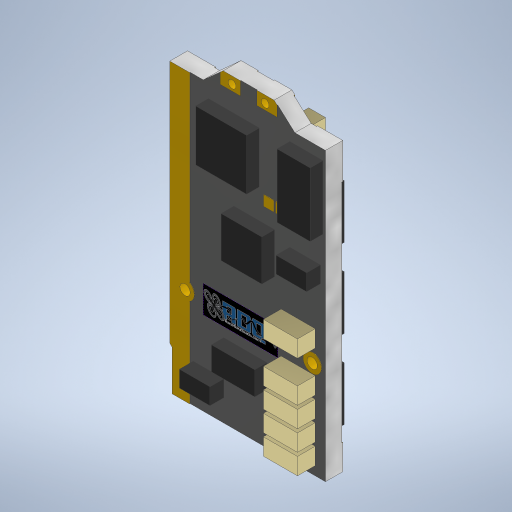
# Autodesk Inventor part: RDQ ESC32
Saved by Autodesk Inventor 2023.1 (Build 271208000, 208)
## iProperties
Created: 2022-10-08
Part Number: RDQ ESC32
Material: GFRC
Document SubType Name: Modeling
Designer: Nathan Cai
Density: 1.7 g/cm^3
Appearance: Flat - Polished Gray
Mass: 3.56 g
Surface Area: 10.1161 cm^2
Volume: 0.696974 cm^3
Author: Nathan Cai
Autodesk Inventor part; units mm, degrees
ref_plane "YZ Plane" through (0, 0, 0) normal (1, 0, 0) x (0, 1, 0)
ref_plane "XZ Plane" through (0, 0, 0) normal (0, 1, 0) x (-1, 0, 0)
ref_plane "XY Plane" through (0, 0, 0) normal (0, 0, 1) x (1, 0, 0)
sketch "Sketch1" plane through (0, 0, 0) normal (0, 0, 1) x (1, 0, 0)
  line L0 (-7.5, 15) -> (7.5, 15)
  line L1 (7.5, 15) -> (7.5, -15)
  line L2 (7.5, -15) -> (-7.5, -15)
  line L3 (-7.5, -15) -> (-7.5, 15)
  line L4 (-7.5, 15) -> (7.5, -15) construction
  line L5 (7.5, 15) -> (-7.5, -15) construction
  line L6 (-7.5, 13.2) -> (7.5, 13.2)
  line L7 (-2.5, 11.4) -> (2.5, 11.4) construction
  line L8 (2.5, 11.4) -> (2.5, 15) construction
  line L9 (2.5, 15) -> (-2.5, 15)
  line L10 (-2.5, 15) -> (-2.5, 11.4) construction
  line L11 (-2.5, 11.4) -> (2.5, 15) construction
  line L12 (2.5, 11.4) -> (-2.5, 15) construction
  line L13 (-4.5, 13.2) -> (-2.5, 15)
  line L14 (2.5, 15) -> (4.5, 13.2)
  line L15 (-4.5, 13.2) -> (4.5, 13.2) construction
  point P0 (0, 0)
  point P1 (0, 13.2)
  dimension "d0" = 15
  dimension "d1" = 30
  dimension "d4" = 28.2
  dimension "d5" = 5
  dimension "d6" = 9
  constraints: 32 end point, 6 midpoint, 5 point on line, 4 parallel, 3 perpendicular, 2 horizontal, 1 collinear
  measures "d0" distance of L1.end L2.end
  measures "d1" distance of L0.end L1.end
  measures "d4" distance between parallel lines of L2 L6
  measures "d5" distance of L9.end L8.end
  measures "d6" distance of L14.end L13.start
extrude "Extrusion1" add sketch "Sketch1" along normal blind 1.6 contours L0 L14 L6 L13 | L6 L1 L2 L3
sketch "Sketch3" plane through (0, 0, 1.6) normal (0, 0, 1) x (1, 0, 0)
  line L0 (2.5, 15) -> (-2.5, 15) projected
  line L1 (-0.8, 15) -> (-2.8, 15)
  line L2 (-2.8, 15) -> (-2.8, 13.7)
  line L3 (-2.8, 13.7) -> (-0.8, 13.7)
  line L4 (-0.8, 13.7) -> (-0.8, 15)
  line L5 (2.5, 15) -> (-2.5, 15) projected
  line L6 (0, 15) -> (0, -15) construction
  line L7 (-7.5, -15) -> (7.5, -15) projected
  line L8 (0.8, 15) -> (2.8, 15)
  line L9 (2.8, 15) -> (2.8, 13.7)
  line L10 (2.8, 13.7) -> (0.8, 13.7)
  line L11 (0.8, 13.7) -> (0.8, 15)
  line L12 (-4.5, 13.2) -> (-7.5, 13.2) projected
  line L13 (-7.5, 13.2) -> (-5.8, 13.2)
  line L14 (-5.8, -15) -> (-7.5, -15)
  line L15 (-7.5, -15) -> (-7.5, 13.2)
  circle A0 centre (-6.25, -5.5) radius 0.5
  circle A1 centre (-6.25, -5.5) radius 0.9
  circle A2 centre (6.25, -5.5) radius 0.5
  circle A3 centre (6.25, -5.5) radius 0.9
  line L16 (-5.8, 13.2) -> (-5.8, -4.7206)
  line L17 (-5.8, -6.2794) -> (-5.8, -15)
  line L18 (1.45, 6.45) -> (2.45, 6.45)
  line L19 (2.45, 6.45) -> (2.45, 5.45)
  line L20 (2.45, 5.45) -> (1.45, 5.45)
  line L21 (1.45, 5.45) -> (1.45, 6.45)
  line L22 (1.45, 6.45) -> (2.45, 5.45) construction
  line L23 (2.45, 6.45) -> (1.45, 5.45) construction
  line L24 (2.65, 5.45) -> (3.65, 5.45)
  line L25 (3.65, 5.45) -> (3.65, 6.45)
  line L26 (3.65, 6.45) -> (2.65, 6.45)
  line L27 (2.65, 6.45) -> (2.65, 5.45)
  line L28 (2.65, 5.45) -> (3.65, 6.45) construction
  line L29 (3.65, 5.45) -> (2.65, 6.45) construction
  line L30 (7.5, 13.2) -> (4.5, 13.2) projected
  line L31 (7.5, -15) -> (7.5, 13.2) projected
  circle A4 centre (-1.625, 14.3) radius 0.375
  circle A5 centre (1.625, 14.3) radius 0.375
  line L32 (-7.5, 13.2) -> (-7.5, -15) projected
  line L33 (-7.5, 13.2) -> (-7.75, 13.2)
  line L34 (-7.75, 13.2) -> (-7.75, -10.8)
  line L35 (-7.75, -10.8) -> (-7.5, -10.8) construction
  line L36 (-7.5, -10.8) -> (-7.5, 13.2)
  line L37 (-7.75, -10.8) -> (-7.4606, -11.0894)
  line L38 (-7.75, -10.8) -> (-7.3407, -10.8) construction
  line L39 (-4.5, 13.2) -> (-2.5, 15)
  line L40 (2.5, 15) -> (4.5, 13.2)
  point P0 (0, 0)
  point P1 (-2.8, 14.35)
  point P2 (1.95, 5.95)
  point P3 (3.15, 5.95)
  point P4 (-7.5, -11.05)
  point P5 (2.8, 14.73)
  point P6 (-2.8, 14.73)
  dimension "d8" = 2
  dimension "d9" = 1.3
  dimension "d10" = 5.6
  dimension "d11" = 1.7
  dimension "d12" = 1
  dimension "d13" = 1.25
  dimension "d14" = 1.8
  dimension "d15" = 9.5
  dimension "d16" = 1
  dimension "d17" = 1
  dimension "d18" = 1
  dimension "d19" = 1
  dimension "d20" = 0.2
  dimension "d21" = 6.75
  dimension "d22" = 3.85
  dimension "d23" = 0.75
  dimension "d24" = 3.25
  dimension "d25" = 0.7
  dimension "d28" = 0.25
  dimension "d29" = 24
  dimension "d30" = 45
  constraints: 68 end point, 11 parallel, 7 midpoint, 7 symmetric about line, 6 centre point, 6 horizontal, 6 perpendicular, 4 point on line, 2 coincident, 2 point on circle, 1 equal length, 3 other
  measures "d8" distance of L3.end L2.end
  measures "d9" distance of L2.end L1.end
  measures "d10" distance from line of point (-2.8, 14.35) L9
  measures "d11" distance of L14.start L14.end
  measures "d12" diameter of A0
  measures "d13" distance from line of L15 A0.centre
  measures "d14" diameter of A1
  measures "d15" distance from line of L7 A1.centre
  measures "d16" distance of L19.end L20.end
  measures "d17" distance of L18.end L19.end
  measures "d18" distance of L26.end L25.end
  measures "d19" distance of L25.end L24.end
  measures "d20" distance between parallel lines of L19 L27
  measures "d21" distance between parallel lines of L30 L26
  measures "d22" distance between parallel lines of L31 L25
  measures "d23" diameter of A4
  measures "d24" distance between centres of A4 A5
  measures "d25" distance from line of L0 A4.centre
  measures "d28" distance of L35.end L34.end
  measures "d29" distance of L34.end L33.end
  measures "d30" angle of L37 L38
extrude "Extrusion2" add sketch "Sketch3" along normal blind 0.05 contours L40 L9 L10 L11 L0 | L4 L3 L2 L39 L0 | L7 L15 L12 L16 A1 L17 | A1 | A3 | L18 L19 L20 L21 | L27 L26 L25 L24
extrude "Extrusion3" add sketch "Sketch3" along normal blind 0.05 and the other way blind 1.6 contours L15 L37 L34 L33
extrude "Extrusion4" cut sketch "Sketch3" against normal through all contours A0 | A2 | A4 | A5
extrude "Extrusion5" add sketch "Sketch3" against normal blind 1.7 contours L40 L9 L10 L11 L0 | L4 L3 L2 L39 L0 | A1 | A3
sketch "Sketch4" plane through (0, 0, 0) normal (0, 0, -1) x (-1, 0, 0)
  line L0 (7.5, -11.05) -> (7.75, -10.8) projected
  line L1 (4.5, 13.2) -> (7.75, 13.2) projected
  line L2 (7.5, -11.05) -> (7.75, -11.05) construction
  line L3 (7.75, -11.05) -> (7.75, 13.2)
  line L4 (7.75, 13.2) -> (7.5, 13.2)
  line L5 (7.5, 13.2) -> (7.5, -11.05)
  line L6 (7.5, -11.05) -> (7.75, -10.8)
  line L7 (-7.5, -15) -> (-7.5, 13.2) projected
  line L8 (-7.5, 13.2) -> (-5, 13.2)
  line L9 (-5, 13.2) -> (-5, 9.7)
  line L10 (-5, 9.7) -> (-7.5, 9.7)
  line L11 (-7.5, 9.7) -> (-7.5, 13.2)
  line L12 (7.5, 13.2) -> (5, 13.2)
  line L13 (5, 13.2) -> (5, 9.7)
  line L14 (5, 9.7) -> (7.5, 9.7)
  line L15 (7.5, 9.7) -> (7.5, 13.2)
  line L16 (-7.5, -15) -> (-4.1, -15)
  line L17 (-4.1, -15) -> (-4.1, -12.5)
  line L18 (-4.1, -12.5) -> (-7.5, -12.5)
  line L19 (-7.5, -12.5) -> (-7.5, -15)
  line L20 (7.5, -15) -> (-7.5, -15) projected
  line L21 (7.5, -15) -> (4, -15)
  line L22 (4, -15) -> (4, -12.5)
  line L23 (4, -12.5) -> (7.5, -12.5)
  line L24 (7.5, -12.5) -> (7.5, -15)
  line L25 (-2.1, -15) -> (1.4, -15)
  line L26 (1.4, -15) -> (1.4, -12.5)
  line L27 (1.4, -12.5) -> (-2.1, -12.5)
  line L28 (-2.1, -12.5) -> (-2.1, -15)
  point P0 (0, 0)
  point P1 (1.4, -15)
  dimension "d39" = 2.5
  dimension "d40" = 3.5
  dimension "d41" = 2.5
  dimension "d42" = 3.5
  dimension "d43" = 3.4
  dimension "d44" = 2.5
  dimension "d45" = 3.5
  dimension "d46" = 2.5
  dimension "d47" = 3.5
  dimension "d48" = 2.5
  dimension "d49" = 2
  constraints: 50 end point, 13 equal length, 6 horizontal, 6 perpendicular, 1 point on line
  measures "d39" distance of L9.end L10.end
  measures "d40" distance of L8.end L9.end
  measures "d41" distance of L14.end L13.end
  measures "d42" distance of L13.end L12.end
  measures "d43" distance of L18.end L17.end
  measures "d44" distance of L17.end L16.end
  measures "d45" distance of L22.end L23.end
  measures "d46" distance of L21.end L22.end
  measures "d47" distance of L27.end L26.end
  measures "d48" distance of L26.end L25.end
  measures "d49" distance between parallel lines of L17 L28
extrude "Extrusion6" add sketch "Sketch4" along normal blind 0.1
sketch "Sketch5" plane through (0, 0, 0) normal (0, 0, -1) x (-1, 0, 0)
  line L0 (-0.75, 8.7) -> (-6.5, 8.7)
  line L1 (-6.5, 8.7) -> (-6.5, 3.45)
  line L2 (-6.5, 3.45) -> (-0.75, 3.45)
  line L3 (-0.75, 3.45) -> (-0.75, 8.7)
  line L4 (-7.5, -12.5) -> (-7.5, 9.7) projected
  line L5 (-7.5, 9.7) -> (-5, 9.7) projected
  line L6 (-0.75, 0.95) -> (-6.5, 0.95)
  line L7 (-6.5, 0.95) -> (-6.5, -4.3)
  line L8 (-6.5, -4.3) -> (-0.75, -4.3)
  line L9 (-0.75, -4.3) -> (-0.75, 0.95)
  line L10 (-0.75, -6.8) -> (-6.5, -6.8)
  line L11 (-6.5, -6.8) -> (-6.5, -12.05)
  line L12 (-6.5, -12.05) -> (-0.75, -12.05)
  line L13 (-0.75, -12.05) -> (-0.75, -6.8)
  line L14 (6, 8.7) -> (0.25, 8.7)
  line L15 (0.25, 8.7) -> (0.25, 3.45)
  line L16 (0.25, 3.45) -> (6, 3.45)
  line L17 (6, 3.45) -> (6, 8.7)
  line L18 (6, 0.95) -> (0.25, 0.95)
  line L19 (0.25, 0.95) -> (0.25, -4.3)
  line L20 (0.25, -4.3) -> (6, -4.3)
  line L21 (6, -4.3) -> (6, 0.95)
  line L22 (6, -6.8) -> (0.25, -6.8)
  line L23 (0.25, -6.8) -> (0.25, -12.05)
  line L24 (0.25, -12.05) -> (6, -12.05)
  line L25 (6, -12.05) -> (6, -6.8)
  line L26 (-1.15, 12.7) -> (2.25, 12.7)
  line L27 (2.25, 12.7) -> (2.25, 9.3)
  line L28 (2.25, 9.3) -> (-1.15, 9.3)
  line L29 (-1.15, 9.3) -> (-1.15, 12.7)
  line L30 (-1.15, 12.7) -> (2.25, 9.3) construction
  line L31 (2.25, 12.7) -> (-1.15, 9.3) construction
  line L32 (7.75, 13.2) -> (5, 13.2) projected
  point P0 (0, 0)
  point P1 (0.55, 11)
  dimension "d52" = 5.25
  dimension "d53" = 5.75
  dimension "d54" = 1
  dimension "d55" = 1
  dimension "d65" = 7.75
  dimension "d68" = 6.75
  dimension "d71" = 3.4
  dimension "d72" = 3.4
  dimension "d73" = 6.35
  dimension "d74" = 0.5
  constraints: 60 end point, 4 parallel, 3 horizontal, 2 collinear, 2 midpoint, 2 perpendicular, 1 vertical, 38 other
  measures "d52" distance between parallel lines of L0 L2
  measures "d53" distance of L1.end L2.end
  measures "d54" distance between parallel lines of L4 L1
  measures "d55" distance between parallel lines of L5 L0
  measures "d65" distance of L0.start L6.start
  measures "d68" distance of L0.start L14.start
  measures "d71" distance of L27.end L28.end
  measures "d72" distance of L26.end L27.end
  measures "d73" distance between parallel lines of L4 L29
  measures "d74" distance between parallel lines of L32 L26
extrude "Extrusion7" add sketch "Sketch5" along normal blind 1.25
sketch "Sketch6" plane through (0, 0, -1.25) normal (0, 0, -1) x (-1, 0, 0)
  line L0 (-1.15, 12.7) -> (2.25, 12.7) projected
  line L1 (0.55, 12.7) -> (0.55, 9.3) construction
  line L2 (-1.15, 9.3) -> (2.25, 9.3) projected
  circle A0 centre (0.55, 11) radius 1.375
  point P0 (0, 0)
  dimension "d77" = 2.75
  constraints: 3 midpoint, 2 end point, 1 centre point
  measures "d77" diameter of A0
extrude "Extrusion8" cut sketch "Sketch6" against normal blind 0.1
chamfer "Chamfer1" distance 0.1 angle 45 1 edges at (0.825, 11, -1.15)
sketch "Sketch7" plane through (0, 0, 0) normal (0, 0, -1) x (-1, 0, 0)
  line L0 (-4.15, 12.65) -> (-2.5, 12.65)
  line L1 (-2.5, 12.65) -> (-2.5, 9.3)
  line L2 (-2.5, 9.3) -> (-4.15, 9.3)
  line L3 (-4.15, 9.3) -> (-4.15, 12.65)
  line L4 (-4.15, 12.65) -> (-2.5, 9.3) construction
  line L5 (-2.5, 12.65) -> (-4.15, 9.3) construction
  line L6 (-7.5, 13.2) -> (-7.5, 9.7) projected
  line L7 (-4.1, 2.95) -> (-0.75, 2.95)
  line L8 (-0.75, 2.95) -> (-0.75, 1.3)
  line L9 (-0.75, 1.3) -> (-4.1, 1.3)
  line L10 (-4.1, 1.3) -> (-4.1, 2.95)
  line L11 (-4.1, 2.95) -> (-0.75, 1.3) construction
  line L12 (-0.75, 2.95) -> (-4.1, 1.3) construction
  line L13 (-7.5, -12.5) -> (-7.5, 9.7) projected
  line L14 (-6.5, 3.45) -> (-0.75, 3.45) projected
  line L15 (-4.1, -4.8) -> (-0.75, -4.8)
  line L16 (-0.75, -4.8) -> (-0.75, -6.45)
  line L17 (-0.75, -6.45) -> (-4.1, -6.45)
  line L18 (-4.1, -6.45) -> (-4.1, -4.8)
  line L19 (-4.1, -4.8) -> (-0.75, -6.45) construction
  line L20 (-0.75, -4.8) -> (-4.1, -6.45) construction
  line L21 (-6.5, -4.3) -> (-0.75, -4.3) projected
  point P0 (0, 0)
  point P1 (-3.325, 10.975)
  point P2 (-1.15, 9.3)
  point P3 (-2.425, 2.125)
  point P4 (-2.425, -5.625)
  dimension "d83" = 1.65
  dimension "d84" = 3.35
  dimension "d85" = 5
  dimension "d86" = 3.35
  dimension "d87" = 1.65
  dimension "d88" = 6.75
  dimension "d89" = 0.5
  dimension "d90" = 3.35
  dimension "d91" = 1.65
  dimension "d92" = 0.5
  constraints: 36 end point, 6 midpoint, 6 parallel, 3 horizontal, 3 perpendicular, 2 point on line
  measures "d83" distance of L1.end L2.end
  measures "d84" distance of L0.end L1.end
  measures "d85" distance between parallel lines of L6 L1
  measures "d86" distance of L8.end L9.end
  measures "d87" distance of L7.end L8.end
  measures "d88" distance between parallel lines of L13 L8
  measures "d89" distance between parallel lines of L14 L7
  measures "d90" distance of L16.end L17.end
  measures "d91" distance of L15.end L16.end
  measures "d92" distance between parallel lines of L21 L15
extrude "Extrusion9" add sketch "Sketch7" along normal blind 1.75
sketch "Sketch8" plane through (0, 0, 1.6) normal (0, 0, 1) x (1, 0, 0)
  line L0 (-4, 6.85) -> (1, 6.85)
  line L1 (1, 6.85) -> (1, 11.85)
  line L2 (1, 11.85) -> (-4, 11.85)
  line L3 (-4, 11.85) -> (-4, 6.85)
  line L4 (-4, 6.85) -> (1, 11.85) construction
  line L5 (1, 6.85) -> (-4, 11.85) construction
  line L6 (-4.5, 13.2) -> (-5.8, 13.2) projected
  line L7 (7.5, -15) -> (7.5, 13.2) projected
  line L8 (-1.5, -0.05) -> (2.5, -0.05)
  line L9 (2.5, -0.05) -> (2.5, 3.95)
  line L10 (2.5, 3.95) -> (-1.5, 3.95)
  line L11 (-1.5, 3.95) -> (-1.5, -0.05)
  line L12 (-1.5, -0.05) -> (2.5, 3.95) construction
  line L13 (2.5, -0.05) -> (-1.5, 3.95) construction
  line L14 (4, 5.95) -> (7.25, 5.95)
  line L15 (7.25, 5.95) -> (7.25, 12.2)
  line L16 (7.25, 12.2) -> (4, 12.2)
  line L17 (4, 12.2) -> (4, 5.95)
  line L18 (4, 5.95) -> (7.25, 12.2) construction
  line L19 (7.25, 5.95) -> (4, 12.2) construction
  line L20 (7.5, 13.2) -> (4.5, 13.2) projected
  point P0 (0, 0)
  point P1 (-1.5, 9.35)
  point P2 (0.5, 1.95)
  point P3 (5.625, 9.075)
  dimension "d95" = 5
  dimension "d96" = 5
  dimension "d97" = 1.35
  dimension "d98" = 6.5
  dimension "d99" = 4
  dimension "d100" = 4
  dimension "d101" = 5
  dimension "d102" = 9.25
  dimension "d103" = 3.25
  dimension "d104" = 6.25
  dimension "d105" = 1
  dimension "d106" = 0.25
  constraints: 36 end point, 6 midpoint, 6 parallel, 3 horizontal, 3 perpendicular
  measures "d95" distance of L2.end L1.end
  measures "d96" distance of L1.end L0.end
  measures "d97" distance between parallel lines of L6 L2
  measures "d98" distance between parallel lines of L7 L1
  measures "d99" distance of L10.end L9.end
  measures "d100" distance of L9.end L8.end
  measures "d101" distance between parallel lines of L7 L9
  measures "d102" distance between parallel lines of L6 L10
  measures "d103" distance of L16.end L15.end
  measures "d104" distance of L15.end L14.end
  measures "d105" distance between parallel lines of L20 L16
  measures "d106" distance between parallel lines of L7 L15
extrude "Extrusion10" add sketch "Sketch8" along normal blind 1.25
sketch "Sketch9" plane through (0, 0, 1.6) normal (0, 0, 1) x (1, 0, 0)
  line L0 (6.5, -14.125) -> (3.15, -14.125)
  line L1 (3.15, -14.125) -> (3.15, -12.475)
  line L2 (3.15, -12.475) -> (6.5, -12.475)
  line L3 (6.5, -12.475) -> (6.5, -14.125)
  line L4 (6.5, -14.125) -> (3.15, -12.475) construction
  line L5 (3.15, -14.125) -> (6.5, -12.475) construction
  line L6 (-5.8, -15) -> (7.5, -15) projected
  line L7 (7.5, -15) -> (7.5, 13.2) projected
  line L8 (6.5, -12.125) -> (3.15, -12.125)
  line L9 (3.15, -12.125) -> (3.15, -10.475)
  line L10 (3.15, -10.475) -> (6.5, -10.475)
  line L11 (6.5, -10.475) -> (6.5, -12.125)
  line L12 (6.5, -12.125) -> (3.15, -10.475) construction
  line L13 (3.15, -12.125) -> (6.5, -10.475) construction
  line L14 (6.5, -10.125) -> (3.15, -10.125)
  line L15 (3.15, -10.125) -> (3.15, -8.475)
  line L16 (3.15, -8.475) -> (6.5, -8.475)
  line L17 (6.5, -8.475) -> (6.5, -10.125)
  line L18 (6.5, -10.125) -> (3.15, -8.475) construction
  line L19 (3.15, -10.125) -> (6.5, -8.475) construction
  line L20 (6.5, -8.125) -> (3.15, -8.125)
  line L21 (3.15, -8.125) -> (3.15, -6.475)
  line L22 (3.15, -6.475) -> (6.5, -6.475)
  line L23 (6.5, -6.475) -> (6.5, -8.125)
  line L24 (6.5, -8.125) -> (3.15, -6.475) construction
  line L25 (3.15, -8.125) -> (6.5, -6.475) construction
  line L26 (3.15, -4.125) -> (6.5, -4.125)
  line L27 (6.5, -4.125) -> (6.5, -2.475)
  line L28 (6.5, -2.475) -> (3.15, -2.475)
  line L29 (3.15, -2.475) -> (3.15, -4.125)
  line L30 (3.15, -4.125) -> (6.5, -2.475) construction
  line L31 (6.5, -4.125) -> (3.15, -2.475) construction
  point P0 (0, 0)
  point P1 (4.825, -13.3)
  point P2 (4.825, -11.3)
  point P3 (4.825, -9.3)
  point P4 (4.825, -7.3)
  point P5 (4.825, -3.3)
  dimension "d109" = 3.35
  dimension "d110" = 1.65
  dimension "d111" = 0.875
  dimension "d112" = 1
  dimension "d115" = 2
  dimension "d120" = 3.35
  dimension "d121" = 1.65
  dimension "d122" = 2.35
  constraints: 60 end point, 4 midpoint, 4 parallel, 2 horizontal, 2 perpendicular, 1 collinear, 1 point on line, 1 vertical, 32 other
  measures "d109" distance of L1.end L2.end
  measures "d110" distance of L0.end L1.end
  measures "d111" distance between parallel lines of L6 L0
  measures "d112" distance between parallel lines of L7 L3
  measures "d115" distance of L0.start L8.start
  measures "d120" distance of L28.end L27.end
  measures "d121" distance of L27.end L26.end
  measures "d122" distance between parallel lines of L22 L26
extrude "Extrusion11" add sketch "Sketch9" along normal blind 1.75
sketch "Sketch10" plane through (0, 0, 1.6) normal (0, 0, 1) x (1, 0, 0)
  line L0 (7, 1.6) -> (4, 1.6)
  line L1 (4, 1.6) -> (4, 3.2)
  line L2 (4, 3.2) -> (7, 3.2)
  line L3 (7, 3.2) -> (7, 1.6)
  line L4 (7, 1.6) -> (4, 3.2) construction
  line L5 (4, 1.6) -> (7, 3.2) construction
  line L6 (7.5, -15) -> (7.5, 13.2) projected
  line L7 (7.5, 13.2) -> (4.5, 13.2) projected
  line L8 (-5.5, -12.85) -> (-2.5, -12.85)
  line L9 (-2.5, -12.85) -> (-2.5, -11.25)
  line L10 (-2.5, -11.25) -> (-5.5, -11.25)
  line L11 (-5.5, -11.25) -> (-5.5, -12.85)
  line L12 (-5.5, -12.85) -> (-2.5, -11.25) construction
  line L13 (-2.5, -12.85) -> (-5.5, -11.25) construction
  line L14 (-5.8, -15) -> (7.5, -15) projected
  point P0 (0, 0)
  point P1 (5.5, 2.4)
  point P2 (-4, -12.05)
  point P3 (-5.5, -12.05)
  dimension "d125" = 3
  dimension "d126" = 1.6
  dimension "d127" = 0.5
  dimension "d128" = 10
  dimension "d131" = 3
  dimension "d132" = 1.6
  dimension "d133" = 3.75
  dimension "d134" = 13
  constraints: 24 end point, 5 midpoint, 4 parallel, 2 horizontal, 2 perpendicular
  measures "d125" distance of L1.end L2.end
  measures "d126" distance of L0.end L1.end
  measures "d127" distance between parallel lines of L6 L3
  measures "d128" distance between parallel lines of L7 L2
  measures "d131" distance of L10.end L9.end
  measures "d132" distance of L9.end L8.end
  measures "d133" distance between parallel lines of L14 L10
  measures "d134" distance from line of L6 point (-5.5, -12.05)
extrude "Extrusion12" add sketch "Sketch10" along normal blind 1.35
sketch "Sketch11" plane through (0, 0, 1.6) normal (0, 0, 1) x (1, 0, 0)
  line L0 (-2.5, -10.05) -> (1.75, -10.05)
  line L1 (1.75, -10.05) -> (1.75, -7.75)
  line L2 (1.75, -7.75) -> (-2.5, -7.75)
  line L3 (-2.5, -7.75) -> (-2.5, -10.05)
  line L4 (-2.5, -10.05) -> (1.75, -7.75) construction
  line L5 (1.75, -10.05) -> (-2.5, -7.75) construction
  line L6 (7.5, -15) -> (7.5, 13.2) projected
  line L7 (-5.8, -15) -> (7.5, -15) projected
  point P0 (0, 0)
  point P1 (-0.375, -8.9)
  dimension "d135" = 4.25
  dimension "d136" = 2.3
  dimension "d137" = 10
  dimension "d138" = 7.25
  constraints: 12 end point, 2 midpoint, 2 parallel, 1 horizontal, 1 perpendicular
  measures "d135" distance of L2.end L1.end
  measures "d136" distance of L1.end L0.end
  measures "d137" distance between parallel lines of L6 L3
  measures "d138" distance between parallel lines of L7 L2
extrude "Extrusion13" add sketch "Sketch11" along normal blind 1.2
sketch "Sketch12" plane through (0, 0, 1.6) normal (0, 0, 1) x (1, 0, 0)
  line L0 (-4.5239, -4.1146) -> (2.8365, -4.1146) construction
  line L1 (2.8365, -4.1146) -> (2.8365, -6.8001) construction
  line L2 (2.8365, -6.8001) -> (-4.5239, -6.8001) construction
  line L3 (-4.5239, -6.8001) -> (-4.5239, -4.1146) construction
  point P0 (0, 0)
  constraints: 2 other
body "Solid1"
